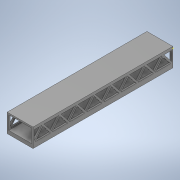
# Autodesk Inventor part: Avionics frame
Saved by Autodesk Inventor 2020.4 (Build 244396000, 396)
## iProperties
Created: 2021-04-27
Part Number: Avionics frame
Material: PC/ABS Plastic
Document SubType Name: Modeling
Designer: armin
Density: 0.357273 g/cm^3
Appearance: Smooth - White
Author: armin
Autodesk Inventor part; units mm, degrees
ref_plane "YZ Plane" through (0, 0, 0) normal (1, 0, 0) x (0, 1, 0)
ref_plane "XZ Plane" through (0, 0, 0) normal (0, 1, 0) x (-1, 0, 0)
ref_plane "XY Plane" through (0, 0, 0) normal (0, 0, 1) x (1, 0, 0)
sketch "Sketch10" plane through (0, 0, 0) normal (0, 1, 0) x (-1, 0, 0)
  point P0 (0, 0)
sketch "Sketch11" plane through (0, 0, 0) normal (0, 1, 0) x (-1, 0, 0)
  line L0 (0, 0) -> (50, 0)
  line L1 (50, 0) -> (50, 270)
  line L2 (50, 270) -> (0, 270)
  line L3 (0, 270) -> (0, 0)
  dimension "d34" = 50
  dimension "d35" = 270
  constraints: 8 end point, 2 parallel, 1 horizontal, 1 perpendicular
  measures "d34" distance of L2.end L1.end
  measures "d35" distance of L1.end L0.end
extrude "Extrusion6" add sketch "Sketch11" along normal blind 3
sketch "Sketch12" plane through (0, 0, 0) normal (0, -1, 0) x (1, 0, 0)
  line L0 (-50, 270) -> (0, 270) projected
  line L1 (-25, 270) -> (-25, 0)
  line L2 (0, 0) -> (-50, 0) projected
  line L3 (-3, 270) -> (-47, 270)
  line L4 (-47, 270) -> (-47, 0)
  line L5 (-47, 0) -> (-3, 0)
  line L6 (-3, 0) -> (-3, 270)
  line L7 (-3, 270) -> (-47, 0) construction
  line L8 (-47, 270) -> (-3, 0) construction
  line L9 (-50, 0) -> (0, 0)
  line L10 (0, 0) -> (0, 270)
  line L11 (0, 270) -> (-50, 270)
  line L12 (-50, 270) -> (-50, 0)
  point P0 (-25, 135)
  point P1 (-3, 0)
  dimension "d38" = 44
  constraints: 22 end point, 5 midpoint, 4 parallel, 2 horizontal, 2 perpendicular, 1 point on line
  measures "d38" distance between parallel lines of L6 L4
extrude "Extrusion7" add sketch "Sketch12" along normal blind 26 contours L0 L4 L2 L12 | L0 L10 L2 L6
sketch "Sketch13" plane through (-50, 3, 0) normal (-1, 0, 0) x (0, 0, 1)
  line L0 (270, -3) -> (270, -29) projected
  line L1 (270, -29) -> (0, -29)
  line L2 (0, -29) -> (0, -3)
  line L3 (0, -3) -> (270, -3)
  line L4 (270, -3) -> (270, -29)
  line L5 (2.5, -26.5) -> (267.5, -26.5)
  line L6 (267.5, -26.5) -> (267.5, -5.5)
  line L7 (267.5, -5.5) -> (2.5, -5.5)
  line L8 (2.5, -5.5) -> (2.5, -26.5)
  line L9 (267.5, -26.5) -> (250.9375, -5.5)
  line L10 (250.9375, -5.5) -> (250.9375, -26.5)
  line L11 (234.375, -26.5) -> (250.9375, -5.5)
  line L12 (265.5896, -26.5) -> (250.9375, -7.9222)
  line L13 (236.2854, -26.5) -> (250.9375, -7.9222)
  line L14 (252.8479, -5.5) -> (267.5, -24.0778)
  line L15 (249.0271, -5.5) -> (232.4646, -26.5)
  line L16 (234.375, -26.5) -> (234.375, -5.5)
  line L17 (232.4646, -26.5) -> (217.8125, -7.9222)
  line L18 (219.7229, -5.5) -> (234.375, -24.0778)
  line L19 (203.1604, -26.5) -> (217.8125, -7.9222)
  line L20 (215.9021, -5.5) -> (199.3396, -26.5)
  line L21 (199.3396, -26.5) -> (184.6875, -7.9222)
  line L22 (186.5979, -5.5) -> (201.25, -24.0778)
  line L23 (170.0354, -26.5) -> (184.6875, -7.9222)
  line L24 (182.7771, -5.5) -> (166.2146, -26.5)
  line L25 (166.2146, -26.5) -> (151.5625, -7.9222)
  line L26 (153.4729, -5.5) -> (168.125, -24.0778)
  line L27 (136.9104, -26.5) -> (151.5625, -7.9222)
  line L28 (149.6521, -5.5) -> (133.0896, -26.5)
  line L29 (133.0896, -26.5) -> (118.4375, -7.9222)
  line L30 (120.3479, -5.5) -> (135, -24.0778)
  line L31 (103.7854, -26.5) -> (118.4375, -7.9222)
  line L32 (116.5271, -5.5) -> (99.9646, -26.5)
  line L33 (99.9646, -26.5) -> (85.3125, -7.9222)
  line L34 (87.2229, -5.5) -> (101.875, -24.0778)
  line L35 (70.6604, -26.5) -> (85.3125, -7.9222)
  line L36 (83.4021, -5.5) -> (66.8396, -26.5)
  line L37 (66.8396, -26.5) -> (52.1875, -7.9222)
  line L38 (54.0979, -5.5) -> (68.75, -24.0778)
  line L39 (37.5354, -26.5) -> (52.1875, -7.9222)
  line L40 (50.2771, -5.5) -> (33.7146, -26.5)
  line L41 (33.7146, -26.5) -> (19.0625, -7.9222)
  line L42 (20.9729, -5.5) -> (35.625, -24.0778)
  line L43 (4.4104, -26.5) -> (19.0625, -7.9222)
  line L44 (17.1521, -5.5) -> (0.5896, -26.5)
  point P0 (2.5, -24.0778)
  point P1 (17.1521, -5.5)
  point P2 (20.9729, -5.5)
  point P3 (35.625, -24.0778)
  point P4 (50.2771, -5.5)
  point P5 (37.5354, -26.5)
  point P6 (66.8396, -26.5)
  point P7 (70.6604, -26.5)
  point P8 (99.9646, -26.5)
  point P9 (54.0979, -5.5)
  point P10 (68.75, -24.0778)
  point P11 (83.4021, -5.5)
  point P12 (87.2229, -5.5)
  point P13 (101.875, -24.0778)
  point P14 (116.5271, -5.5)
  point P15 (120.3479, -5.5)
  point P16 (135, -24.0778)
  point P17 (149.6521, -5.5)
  point P18 (103.7854, -26.5)
  point P19 (136.9104, -26.5)
  point P20 (153.4729, -5.5)
  point P21 (168.125, -24.0778)
  point P22 (182.7771, -5.5)
  point P23 (186.5979, -5.5)
  point P24 (201.25, -24.0778)
  point P25 (215.9021, -5.5)
  point P26 (234.375, -24.0778)
  point P27 (219.7229, -5.5)
  point P28 (99.9646, -26.5)
  dimension "d41" = 2.5
  dimension "d42" = 265
  dimension "d43" = 1.5
  dimension "d45" = 1.5
  dimension "d46" = 1.5
  dimension "d47" = 33.125
  dimension "d50" = 33.125
  constraints: 86 end point, 49 horizontal alignment, 32 parallel, 6 point on line, 2 horizontal, 2 perpendicular, 2 symmetric about line, 2 vertical, 9 other
  measures "d42" distance of L8.end L6.start
  measures "d43" distance between parallel lines of L12 L9
  measures "d45" distance between parallel lines of L9 L14
  measures "d46" distance between parallel lines of L15 L11
  measures "d47" distance between parallel lines of L6 L16
  measures "d50" distance of L12.start L17.start
extrude "Extrusion9" cut sketch "Sketch13" against normal through all contours L43 L41 L5 | L8 L7 L44 | L39 L37 L5 | L42 L7 L40 | L35 L33 L5 | L38 L7 L36 | L31 L29 L5 | L34 L7 L32 | L27 L25 L5 | L30 L7 L28 | L23 L21 L5 | L26 L7 L24 | L19 L17 L5 | L22 L7 L20 | L16 L7 L15 | L18 L7 L16 | L13 L10 L5 | L10 L12 L5 | L7 L6 L14
sketch "Sketch14" plane through (0, -26, 0) normal (0, -1, 0) x (1, 0, 0)
  line L0 (0, 0) -> (-50, 0)
  line L1 (-50, 0) -> (-50, 270)
  line L2 (-50, 270) -> (0, 270)
  line L3 (0, 270) -> (0, 0)
  constraints: 8 end point, 2 parallel, 1 horizontal, 1 perpendicular
extrude "Extrusion10" add sketch "Sketch14" along normal blind 2
sketch "Sketch15" plane through (0, -28, 0) normal (0, -1, 0) x (1, 0, 0)
  line L0 (-50, 0) -> (-50, 270) projected
  line L1 (-50, 135) -> (0, 135)
  line L2 (-3, 0) -> (-3, 270) projected
  line L3 (-47, 3) -> (-3, 3)
  line L4 (-3, 3) -> (-3, 267)
  line L5 (-3, 267) -> (-47, 267)
  line L6 (-47, 267) -> (-47, 3)
  line L7 (-47, 3) -> (-3, 267) construction
  line L8 (-3, 3) -> (-47, 267) construction
  line L9 (0, 270) -> (-50, 270) projected
  line L10 (0, 270) -> (0, 0) projected
  line L11 (-50, 270) -> (0, 270)
  line L12 (0, 270) -> (0, 0)
  line L13 (0, 0) -> (-50, 0)
  line L14 (-50, 0) -> (-50, 270)
  line L15 (-50, 270) -> (0, 0) construction
  line L16 (0, 270) -> (-50, 0) construction
  point P0 (-25, 135)
  dimension "d61" = 3
  dimension "d62" = 3
  dimension "d65" = 0
  constraints: 26 end point, 6 midpoint, 4 parallel, 3 perpendicular, 2 horizontal
  measures "d61" distance between parallel lines of L5 L9
  measures "d62" distance between parallel lines of L6 L0
  measures "d65" distance between parallel lines of L0 L14
extrude "Extrusion11" add sketch "Sketch15" along normal blind 5 contours L0 L1 L6 L3 L2 L13 | L0 L9 L2 L5 L6 L1 | L2 L1 L10 L13 | L9 L10 L1 L2
equation "\"d47\" = 0.125 * d42"
body "Solid2"
